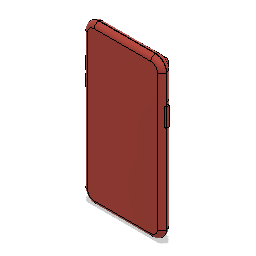
IPHONE_11P (PENDING CHECK) v4 (Autodesk Fusion 360 design; units mm, degrees)
Autodesk Fusion 360 part; units mm, degrees
sketch "Sketch1" plane through (0, 0, 0) normal (0, 0, 1) x (1, 0, 0)
  line L0 (35.7, 72) -> (-35.7, 72)
  line L1 (-35.7, 72) -> (-35.7, -72)
  line L2 (-35.7, -72) -> (35.7, -72)
  line L3 (35.7, -72) -> (35.7, 72)
  line L4 (35.7, 72) -> (-35.7, -72) construction
  line L5 (-35.7, 72) -> (35.7, -72) construction
  dimension "d1" = 71.4
  dimension "d2" = 144
  constraint horizontal L0
  constraint perpendicular L0 L1
  constraint parallel L0 L2
  constraint parallel L1 L3
  constraint coincident L4 origin
  constraint coincident L5 origin
  measures "d1" distance of L1.end L2.end
  measures "d2" distance of L0.end L1.end
extrude "Extrude1" add sketch "Sketch1" along normal blind 8.3 makes body 1
sketch "Sketch3" plane through (0, 0, 0) normal (0, 0, -1) x (1, 0, 0)
  line L0 (3.2, -37) -> (32.2, -37)
  line L1 (32.2, -37) -> (32.2, -68)
  line L2 (32.2, -68) -> (3.2, -68)
  line L3 (3.2, -68) -> (3.2, -37)
  line L4 (3.2, -37) -> (32.2, -68) construction
  line L5 (32.2, -37) -> (3.2, -68) construction
  line L6 (-35.7, 72) -> (-35.7, -72)
  line L7 (-35.7, -72) -> (35.7, -72)
  line L8 (35.7, -72) -> (35.7, 72)
  line L9 (35.7, 72) -> (-35.7, 72)
  point P0 (17.7, -52.5)
  dimension "d9" = 29
  dimension "d10" = 31
  dimension "d31" = 4
  dimension "d32" = 3.5
  constraint horizontal L0
  constraint perpendicular L0 L1
  constraint parallel L0 L2
  constraint parallel L1 L3
  constraint coincident L4 P0
  constraint coincident L5 P0
  measures "d9" distance of L0.start L0.end
  measures "d10" distance of L0.start L2.end
  measures "d31" distance of L2 L7
  measures "d32" distance of L1 L8
extrude "Extrude2" add sketch "Sketch3" along normal blind 1.25 contours L0 L1 L2 L3 bodies 1
fillet "Fillet2" radius 3 4 edges at (32.2, 68, -0.625) (32.2, 37, -0.625) (3.2, 68, -0.625) (3.2, 37, -0.625) on bodies 1
sketch "Sketch4" plane through (35.7, 0, 0) normal (1, 0, 0) x (0, 0, -1)
  line L0 (0, -72) -> (0, 72)
  line L1 (-8.3, 72) -> (-8.3, -72)
  line L2 (1.25, 40) -> (1.25, 37)
  line L3 (1.25, 37) -> (0, 37)
  line L4 (1.25, 40) -> (1.25, 65)
  line L5 (1.25, 68) -> (1.25, 65)
  line L6 (0, 68) -> (1.25, 68)
  line L7 (0, 72) -> (0, 68)
  line L8 (-8.3, 72) -> (-8.3, -72)
  line L9 (-4.15, 72) -> (-4.15, -72) construction
  line L10 (-2.9, 19) -> (-5.4, 19)
  line L11 (-5.4, 19) -> (-5.4, 36)
  line L12 (-5.4, 36) -> (-2.9, 36)
  line L13 (-2.9, 36) -> (-2.9, 19)
  line L14 (-2.9, 19) -> (-5.4, 36) construction
  line L15 (-5.4, 19) -> (-2.9, 36) construction
  line L16 (0, 72) -> (-8.3, 72)
  line L17 (-8.3, -72) -> (0, -72)
  line L18 (0, -72) -> (-8.3, -72)
  line L19 (0, 72) -> (-8.3, 72)
  line L20 (0, 37) -> (0, -72)
  point P0 (-4.15, 27.5)
  dimension "d20" = 2.5
  dimension "d21" = 17
  dimension "d33" = 36
  constraint horizontal L10
  constraint perpendicular L10 L11
  constraint parallel L10 L12
  constraint parallel L11 L13
  constraint coincident L14 P0
  constraint coincident L15 P0
  constraint coincident L9 P0
  constraint midpoint L9.end L17
  constraint perpendicular L9 L17
  constraint midpoint L9.start L19
  measures "d20" distance of L10.start L10.end
  measures "d21" distance of L10.start L12.end
  measures "d33" distance of L12 L19
extrude "Extrude3" add sketch "Sketch4" along normal blind 1 contours L10 L11 L12 L13 bodies 1
sketch "Sketch5" plane through (-35.7, 0, 0) normal (-1, 0, 0) x (0, 0, 1)
  line L0 (8.3, -72) -> (8.3, 72)
  line L1 (0, 72) -> (0, -72)
  line L2 (-1.25, 65) -> (-1.25, 68)
  line L3 (-1.25, 65) -> (-1.25, 40)
  line L4 (-1.25, 37) -> (-1.25, 40)
  line L5 (0, 37) -> (-1.25, 37)
  line L6 (-1.25, 68) -> (0, 68)
  line L7 (0, -72) -> (0, 37)
  line L8 (8.3, -72) -> (8.3, 72)
  line L9 (4.15, 72) -> (4.15, -72) construction
  line L10 (5.4, 28.75) -> (2.9, 28.75)
  line L11 (2.9, 28.75) -> (2.9, 39.5)
  line L12 (2.9, 39.5) -> (5.4, 39.5)
  line L13 (5.4, 39.5) -> (5.4, 28.75)
  line L14 (5.4, 28.75) -> (2.9, 39.5) construction
  line L15 (2.9, 28.75) -> (5.4, 39.5) construction
  line L16 (0, 27.25) -> (8.3, 27.25) construction
  line L17 (2.9, 25.75) -> (2.9, 15)
  line L18 (2.9, 15) -> (5.4, 15)
  line L19 (5.4, 25.75) -> (2.9, 25.75)
  line L20 (5.4, 15) -> (5.4, 25.75)
  line L21 (0, -72) -> (8.3, -72)
  line L22 (8.3, 72) -> (0, 72)
  line L23 (0, -72) -> (8.3, -72)
  line L24 (0, 72) -> (8.3, 72)
  line L25 (0, 68) -> (0, 72)
  point P0 (4.15, 34.125)
  dimension "d25" = 1.5
  dimension "d26" = 10.75
  dimension "d27" = 2.5
  dimension "d38" = 32.5
  constraint horizontal L10
  constraint perpendicular L10 L11
  constraint parallel L10 L12
  constraint parallel L11 L13
  constraint coincident L14 P0
  constraint coincident L15 P0
  constraint coincident L9 P0
  constraint coincident L7 L16.start
  constraint coincident L8 L16.end
  constraint perpendicular L8 L16
  constraint symmetric L10.start L16 L19.start
  constraint symmetric L10.end L16 L17.start
  constraint symmetric L11.end L16 L17.end
  constraint symmetric L12.end L16 L18.end
  constraint midpoint L9.start L22
  constraint perpendicular L9 L22
  constraint midpoint L9.end L23
  measures "d25" distance of L10 L16
  measures "d26" distance of L10.start L12.end
  measures "d27" distance of L10.start L10.end
  measures "d38" distance of L12 L22
extrude "Extrude4" add sketch "Sketch5" along normal blind 1 contours L10 L11 L12 L13 | L17 L18 L19 L20 bodies 1
fillet "Fillet1" radius 10 4 edges at (-35.7, 72, 4.15) (35.7, 72, 4.15) (35.7, -72, 4.15) (-35.7, -72, 4.15) on bodies 1
fillet "Fillet4" radius 4 16 edges at (-32.7711, 69.0711, 0) (-35.7, 0, 0) (-32.7711, -69.0711, 0) (0, -72, 0) (32.7711, -69.0711, 0) (35.7, 0, 0) (32.7711, 69.0711, 0) (0, 72, 0) (35.7, 0, 8.3) (32.7711, -69.0711, 8.3) (0, -72, 8.3) (-32.7711, -69.0711, 8.3) (-35.7, 0, 8.3) (-32.7711, 69.0711, 8.3) (0, 72, 8.3) (32.7711, 69.0711, 8.3) on bodies 1
copy_body "CopyPasteBodies1" bodies 1 makes body 2
move_body "Move1" bodies 2 to x (1, 0, 0) y (0, 1, 0) z (0, 0, 1) at (0, 0, 0)
scale "Scale1" factors (1.006, 1.003, 1.051) about (6.2, 37, 0) bodies 2
copy_body "CopyPasteBodies2" bodies 2 makes body 3
move_body "Move2" bodies 3 to x (-1, 0, 0) y (0, -1, 0) z (0, 0, 1) at (0.0744, -0.228, 0)
hidden bodies 1 3
equation "d25 = ( 3 / 2 ) * 1 mm"
named bodies: "IPHONE_11", "IPHONE_14P", "IPHONE_11_FIT", "IPHONE_14P_FIT", "IPHONE_11_FIT REVERSED"
